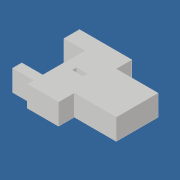
# Autodesk Inventor part: P1704_004_gachette
Saved by Autodesk Inventor 2019 (Build 230136000, 136)
## iProperties
Created: 2019-04-30
Part Number: P1704_004_gachette
Material: Générique
Document SubType Name: Modeling
Designer: Joan.MAILLARD
Density: 1 g/cm^3
Appearance: Par défaut
Author: Joan.MAILLARD
Autodesk Inventor part; units mm, degrees
ref_plane "YZ Plane" through (0, 0, 0) normal (1, 0, 0) x (0, 1, 0)
ref_plane "XZ Plane" through (0, 0, 0) normal (0, 1, 0) x (-1, 0, 0)
ref_plane "XY Plane" through (0, 0, 0) normal (0, 0, 1) x (1, 0, 0)
sketch "Esquisse2" plane through (0, 0, 0) normal (1, 0, 0) x (0, 1, 0)
  line L0 (-5, 10) -> (5, 10)
  line L1 (5, -10) -> (-5, -10)
  line L2 (-5, -10) -> (-5, 10)
  line L3 (-5, 10) -> (5, -10) construction
  line L4 (5, 10) -> (-5, -10) construction
  line L5 (5, -10) -> (5, 10)
  point P0 (0, 0)
  dimension "d2" = 20
  dimension "d7" = 10
  constraints: 12 end point, 2 midpoint, 2 parallel, 1 horizontal, 1 vertical
  measures "d2" distance of L1.end L0.start
  measures "d7" distance of L1.start L1.end
extrude "Extrusion1" add sketch "Esquisse2" along normal blind 20
sketch "Esquisse3" plane through (0, 0, 0) normal (-1, 0, 0) x (0, 0, 1)
  line L0 (-17.5, -5) -> (17.5, -5)
  line L1 (17.5, -5) -> (17.5, 5)
  line L2 (17.5, 5) -> (-17.5, 5)
  line L3 (-17.5, 5) -> (-17.5, -5)
  line L4 (-17.5, -5) -> (17.5, 5) construction
  line L5 (17.5, -5) -> (-17.5, 5) construction
  point P0 (0, 0)
  point P1 (-10, 5)
  dimension "d8" = 35
  constraints: 12 end point, 2 midpoint, 2 parallel, 1 horizontal, 1 perpendicular, 1 point on line
  measures "d8" distance between parallel lines of L1 L3
extrude "Extrusion2" add sketch "Esquisse3" along normal blind 25
sketch "Esquisse4" plane through (-25, 0, 0) normal (-1, 0, 0) x (0, 0, 1)
  line L0 (-10, -5) -> (-10, 5) projected
  line L1 (10, -5) -> (17.5, -5) projected
  line L2 (-10, 5) -> (10, 5)
  line L3 (10, 5) -> (10, -5)
  line L4 (10, -5) -> (-10, -5)
  line L5 (-10, -5) -> (-10, 5)
  point P0 (0, 0)
  constraints: 8 end point, 2 parallel, 1 horizontal, 1 perpendicular
extrude "Extrusion3" cut sketch "Esquisse4" against normal blind 10
sketch "Esquisse6" plane through (20, 5, 10) normal (0, 1, 0) x (1, 0, 0)
  line L0 (-20, -7.5) -> (-20, 0) construction
  line L1 (-35, 27.5) -> (-20, 27.5) construction
  line L2 (-20, 27.5) -> (-20, -7.5) construction
  line L3 (-20, -7.5) -> (-35, -7.5) construction
  line L4 (-35, -7.5) -> (-35, 27.5) construction
  line L5 (-35, 27.5) -> (-20, -7.5) construction
  line L6 (-20, 27.5) -> (-35, -7.5) construction
  line L7 (-30, 11) -> (-25, 11)
  line L8 (-25, 11) -> (-25, 9)
  line L9 (-25, 9) -> (-30, 9)
  line L10 (-30, 9) -> (-30, 11)
  line L11 (-30, 11) -> (-25, 9) construction
  line L12 (-25, 11) -> (-30, 9) construction
  point P0 (-20, 10)
  point P1 (-27.5, 10)
  point P2 (-35, 0)
  dimension "d15" = 2
  dimension "d16" = 5
  constraints: 24 end point, 4 midpoint, 4 parallel, 2 horizontal, 2 perpendicular, 1 coincident, 1 point on line
  measures "d15" distance of L7.end L8.end
  measures "d16" distance of L8.end L9.end
extrude "Extrusion6" cut sketch "Esquisse6" against normal blind 10
sketch "Esquisse8" plane through (-15, 0, 0) normal (-1, 0, 0) x (0, 0, 1)
  point P0 (0, 0)
  point P1 (0, 0)
  constraints: 1 coincident
hole "Perçage1" at (-15, 0, 0) direction (1, 0, 0) diameter 3 depth 10
sketch "Esquisse9" plane through (-25, 0, 0) normal (-1, 0, 0) x (0, 0, 1)
  line L0 (17.5, 5) -> (14.5, 5)
  line L1 (14.5, 5) -> (14.5, -5)
  line L2 (14.5, -5) -> (17.5, -5)
  line L3 (17.5, -5) -> (17.5, 5)
  line L4 (10, -5) -> (17.5, -5) projected
  dimension "d31" = 3
  constraints: 8 end point, 2 parallel, 1 coincident, 1 horizontal, 1 perpendicular, 1 point on line
  measures "d31" distance between parallel lines of L3 L1
extrude "Extrusion8" cut sketch "Esquisse9" against normal blind 10
